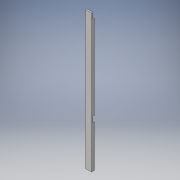
# Autodesk Inventor part: Cabinet Support Frame Center Vertical Bar
Saved by Autodesk Inventor 2016 (Build 200138000, 138)
## iProperties
Created: 2018-02-03
Part Number: Cabinet Support Frame Center Vertical Bar
Material: Generic
Document SubType Name: Modeling
Designer: dash
Density: 1 g/cm^3
Appearance: Default
Author: dash
Autodesk Inventor part; units mm, degrees
ref_plane "YZ Plane" through (0, 0, 0) normal (1, 0, 0) x (0, 1, 0)
ref_plane "XZ Plane" through (0, 0, 0) normal (0, 1, 0) x (-1, 0, 0)
ref_plane "XY Plane" through (0, 0, 0) normal (0, 0, 1) x (1, 0, 0)
sketch "Sketch1" plane through (0, 0, 0) normal (0, 0, 1) x (1, 0, 0)
  line L0 (657.7721, 961.825) -> (695.8721, 961.825)
  line L1 (695.8721, 961.825) -> (695.8721, 82.35)
  line L2 (695.8721, 82.35) -> (657.7721, 82.35)
  line L3 (657.7721, 82.35) -> (657.7721, 961.825)
  point P0 (0, 0)
  dimension "d0" = 879.475
  dimension "d1" = 38.1
  constraints: 8 end point, 2 parallel, 1 horizontal, 1 perpendicular
  measures "d0" distance of L0.end L1.end
  measures "d1" distance of L1.end L2.end
extrude "Board" add sketch "Sketch1" along normal blind 19.05
sketch "Sketch2" plane through (0, 0, 0) normal (0, 0, -1) x (-1, 0, 0)
  line L0 (-695.8721, 82.35) -> (-695.8721, 961.825) projected
  line L1 (-657.7721, 961.825) -> (-657.7721, 82.35) projected
  line L2 (-695.8721, 961.825) -> (-657.7721, 961.825)
  line L3 (-657.7721, 961.825) -> (-657.7721, 923.725)
  line L4 (-657.7721, 923.725) -> (-695.8721, 923.725)
  line L5 (-695.8721, 923.725) -> (-695.8721, 961.825)
  point P0 (0, 0)
  dimension "d4" = 38.1
  constraints: 8 end point, 2 parallel, 1 horizontal, 1 perpendicular, 1 point on line
  measures "d4" distance of L2.end L3.end
extrude "Top Notch" cut sketch "Sketch2" against normal blind 9.525
sketch "Sketch3" plane through (0, 0, 0) normal (0, 0, -1) x (-1, 0, 0)
  line L0 (-695.8721, 923.725) -> (-695.8721, 82.35) projected
  line L1 (-657.7721, 961.825) -> (-657.7721, 82.35) projected
  line L2 (-695.8721, 387.15) -> (-657.7721, 387.15)
  line L3 (-657.7721, 387.15) -> (-657.7721, 349.05)
  line L4 (-657.7721, 349.05) -> (-695.8721, 349.05)
  line L5 (-695.8721, 349.05) -> (-695.8721, 387.15)
  line L6 (-695.8721, 82.35) -> (-657.7721, 82.35) projected
  line L7 (-695.8721, 961.825) -> (-657.7721, 961.825) projected
  point P0 (0, 0)
  dimension "d7" = 38.1
  dimension "d11" = 574.675
  constraints: 8 end point, 2 parallel, 2 point on line, 1 horizontal, 1 perpendicular
  measures "d7" distance between parallel lines of L4 L2
  measures "d11" distance between parallel lines of L2 L7
extrude "Bottom Notch" cut sketch "Sketch3" against normal blind 9.525 contours L2 L1 L4 L0
body "Solid1"
